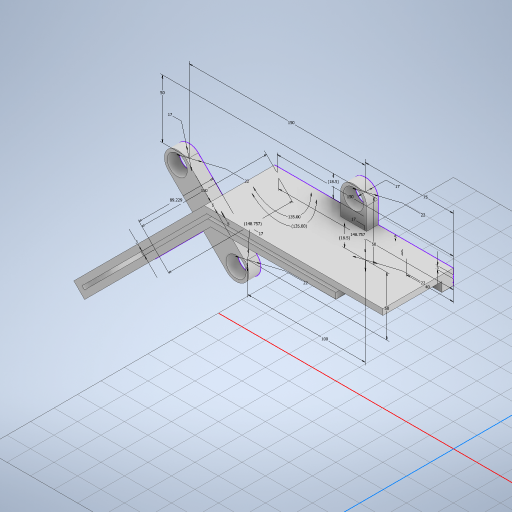
# Autodesk Inventor part: hold_left
Saved by Autodesk Inventor 2024 (Build 280153000, 153)
## iProperties
Created: 2024-02-27
Part Number: hold_left
Material: Generic
Document SubType Name: Modeling
Designer: Administrator
Density: 1 g/cm^3
Appearance: Default
Author: Administrator
Autodesk Inventor part; units mm, degrees
ref_plane "YZ Plane" through (0, 0, 0) normal (1, 0, 0) x (0, 1, 0)
ref_plane "XZ Plane" through (0, 0, 0) normal (0, 1, 0) x (-1, 0, 0)
ref_plane "XY Plane" through (0, 0, 0) normal (0, 0, 1) x (1, 0, 0)
sketch "Sketch1" plane through (0, 0, 0) normal (0, 0, 1) x (1, 0, 0)
  line L0 (-150, 1.5) -> (-256.066, -104.566)
  line L1 (-256.066, -104.566) -> (-253.9447, -106.6873)
  line L2 (-253.9447, -106.6873) -> (-148.7574, -1.5)
  line L3 (0, 1.5) -> (0, -1.5)
  line L4 (0, -1.5) -> (-148.7574, -1.5)
  line L5 (-150, 1.5) -> (0, 1.5)
  line L6 (-263.1371, -104.566) -> (-152.0711, 6.5)
  line L7 (-152.0711, 6.5) -> (0, 6.5)
  line L8 (0, -6.5) -> (-146.6863, -6.5)
  line L9 (-146.6863, -6.5) -> (-253.9447, -113.7584)
  line L10 (-253.9447, -113.7584) -> (-263.1371, -104.566)
  line L11 (0, 1.5) -> (0, 6.5)
  line L12 (0, -1.5) -> (0, -6.5)
  circle A0 centre (-75, 25) radius 11
  circle A1 centre (-175, -75) radius 11
  circle A2 centre (-75, -25) radius 11
  circle A3 centre (-225, -25) radius 11
  line L13 (-232.7782, -32.7782) -> (-212.0637, -53.4926)
  line L14 (-182.7782, -82.7782) -> (-202.8713, -62.685)
  line L15 (-167.2218, -67.2218) -> (-187.315, -47.1287)
  line L16 (-86, 25) -> (-86, 6.5)
  line L17 (-64, 25) -> (-64, 6.5)
  line L18 (-217.2218, -17.2218) -> (-196.5074, -37.9363)
  line L19 (-40, -1.5) -> (-40, -6.5)
  line L20 (-86, -25) -> (-86, -6.5)
  line L21 (-64, -25) -> (-64, -6.5)
  circle A4 centre (-75, 25) radius 8.5
  circle A5 centre (-75, -25) radius 8.5
  circle A6 centre (-175, -75) radius 8.5
  circle A7 centre (-225, -25) radius 8.5
  point P0 (0, 0)
  point P1 (0, 0)
  point P2 (-76.0355, 6.5)
  point P3 (0, -4)
  dimension "d2" = 150
  dimension "d4" = 3
  dimension "d5" = 3
  dimension "d6" = 135
  dimension "d7" = 150
  dimension "d8" = 148.7574
  dimension "d9" = 135
  dimension "d10" = 148.7574
  dimension "d11" = 5
  dimension "d12" = 5
  dimension "d13" = 5
  dimension "d14" = 5
  dimension "d31" = 22
  dimension "d33" = 22
  dimension "d39" = 75
  dimension "d41" = 22
  dimension "d42" = 50
  dimension "d47" = 22
  dimension "d57" = 18.5
  dimension "d60" = 18.5
  dimension "d62" = 150
  dimension "d63" = 50
  dimension "d64" = 100
  dimension "d65" = 50
  dimension "d66" = 40
  dimension "d70" = 17
  dimension "d71" = 17
  dimension "d72" = 17
  dimension "d73" = 17
  dimension "d78" = 89.2287
  constraints: 44 end point, 11 point on line, 10 perpendicular, 8 centre point, 8 point on circle, 6 tangent, 4 coincident, 3 midpoint, 3 parallel, 1 horizontal, 1 other
  measures "d2" distance of L0.start L0.end
  measures "d4" distance of L0.end L1.end
  measures "d5" distance of L3.start L3.end
  measures "d6" angle of L4 L2
  measures "d7" distance of L0.start L3.start
  measures "d8" distance of L3.end L2.end
  measures "d9" angle of L5 L0
  measures "d10" distance of L1.end L2.end
  measures "d11" distance between parallel lines of L0 L6
  measures "d12" distance between parallel lines of L7 L5
  measures "d13" distance between parallel lines of L4 L8
  measures "d14" distance between parallel lines of L9 L2
  measures "d31" diameter of A0
  measures "d33" diameter of A1
  measures "d39" horizontal distance of L3.start A0.centre
  measures "d41" diameter of A2
  measures "d42" distance of A2.centre A0.centre
  measures "d47" diameter of A3
  measures "d57" distance from line of L8 A2.centre
  measures "d60" vertical distance of point (-76.036, 6.5) A0.centre
  measures "d62" horizontal distance of A0.centre A3.centre
  measures "d63" vertical distance of A0.centre A3.centre
  measures "d64" horizontal distance of A2.centre A1.centre
  measures "d65" vertical distance of A2.centre A1.centre
  measures "d66" distance from line of point (0, -4) L19
  measures "d70" diameter of A4
  measures "d71" diameter of A5
  measures "d72" diameter of A6
  measures "d73" diameter of A7
  measures "d78" distance between parallel lines of L15 L1
extrude "Extrusion2" add sketch "Sketch1" along normal blind 10 contours L5 L3 L4 L2 L1 L0 | L12 L8 L19 L4 | L7 L16 A0 L17 | A0 | L21 A2 L20 L8 | A2 | L6 L13 A3 L18 | A3 | L15 A1 L14 L9 | A1
extrude "Extrusion3" add sketch "Sketch1" along normal blind 60 contours L0 L1 L2 L4 L19 L8 L9 L10 L6 L7 L11 L5
body "Solid1"
